Autodesk Fusion 360 part; units mm, degrees
(part 5 of 7)
  spline S636 degree 3 poles (-2.5533, 4.7746) (-2.5168, 4.7495) (-2.4648, 4.7165) (-2.4379, 4.7009) knots 0 0 0 0 1 1 1 1
  spline S637 degree 3 poles (-2.4379, 4.7009) (-2.4119, 4.6862) (-2.3824, 4.6662) (-2.3737, 4.6567) knots 0 0 0 0 1 1 1 1
  spline S638 degree 3 poles (-2.3737, 4.6567) (-2.359, 4.6393) (-2.359, 4.6385) (-2.3789, 4.622) knots 0 0 0 0 1 1 1 1
  spline S639 degree 3 poles (-2.3789, 4.622) (-2.391, 4.6116) (-2.3945, 4.6046) (-2.3884, 4.6038) knots 0 0 0 0 1 1 1 1
  spline S640 degree 3 poles (-2.3884, 4.6038) (-2.3824, 4.6038) (-2.3798, 4.5994) (-2.3832, 4.5942) knots 0 0 0 0 1 1 1 1
  spline S641 degree 3 poles (-2.3832, 4.5942) (-2.3867, 4.5873) (-2.4049, 4.5864) (-2.4353, 4.5899) knots 0 0 0 0 1 1 1 1
  line L91 (-2.4353, 4.5899) -> (-2.4821, 4.5951)
  line L92 (-2.4821, 4.5951) -> (-2.5411, 4.5413)
  spline S642 degree 3 poles (-2.5411, 4.5413) (-2.5732, 4.5118) (-2.6981, 4.3878) (-2.8187, 4.2663) knots 0 0 0 0 1 1 1 1
  spline S643 degree 3 poles (-2.8187, 4.2663) (-2.9661, 4.1171) (-3.0373, 4.0391) (-3.0373, 4.0261) knots 0 0 0 0 1 1 1 1
  spline S644 degree 3 poles (-3.0373, 4.0261) (-3.0373, 4.0018) (-2.9028, 3.8404) (-2.7875, 3.7277) knots 0 0 0 0 1 1 1 1
  spline S645 degree 3 poles (-2.7875, 3.7277) (-2.7363, 3.6773) (-2.6686, 3.608) (-2.6374, 3.5741) knots 0 0 0 0 1 1 1 1
  spline S646 degree 3 poles (-2.6374, 3.5741) (-2.6027, 3.5377) (-2.555, 3.4978) (-2.5168, 3.4752) knots 0 0 0 0 1 1 1 1
  line L93 (-2.5168, 3.4752) -> (-2.4535, 3.4379)
  line L94 (-2.4535, 3.4379) -> (-2.3485, 3.4379)
  spline S647 degree 3 poles (-2.3485, 3.4379) (-2.2774, 3.4388) (-2.228, 3.4431) (-2.1967, 3.4536) knots 0 0 0 0 1 1 1 1
  spline S648 degree 3 poles (-2.1967, 3.4536) (-2.1707, 3.4614) (-2.1308, 3.4674) (-2.1074, 3.4674) knots 0 0 0 0 1 1 1 1
  spline S649 degree 3 poles (-2.1074, 3.4674) (-2.0848, 3.4674) (-2.0432, 3.4752) (-2.0155, 3.4848) knots 0 0 0 0 1 1 1 1
  spline S650 degree 3 poles (-2.0155, 3.4848) (-1.9851, 3.4952) (-1.94, 3.503) (-1.901, 3.503) knots 0 0 0 0 1 1 1 1
  spline S651 degree 3 poles (-1.901, 3.503) (-1.8654, 3.5039) (-1.8012, 3.5099) (-1.7578, 3.5169) knots 0 0 0 0 1 1 1 1
  spline S652 degree 3 poles (-1.7578, 3.5169) (-1.6173, 3.5394) (-1.5904, 3.5412) (-1.5713, 3.5238) knots 0 0 0 0 1 1 1 1
  spline S653 degree 3 poles (-1.5713, 3.5238) (-1.5514, 3.5056) (-1.5488, 3.477) (-1.5653, 3.457) knots 0 0 0 0 1 1 1 1
  spline S654 degree 3 poles (-1.5653, 3.457) (-1.5705, 3.4501) (-1.6008, 3.4301) (-1.6321, 3.4137) knots 0 0 0 0 1 1 1 1
  spline S655 degree 3 poles (-1.6321, 3.4137) (-1.6633, 3.3972) (-1.7223, 3.3633) (-1.7639, 3.3391) knots 0 0 0 0 1 1 1 1
  spline S656 degree 3 poles (-1.7639, 3.3391) (-1.8047, 3.3156) (-1.848, 3.2931) (-1.8593, 3.2896) knots 0 0 0 0 1 1 1 1
  spline S657 degree 3 poles (-1.8593, 3.2896) (-1.8697, 3.2861) (-1.8992, 3.2705) (-1.9235, 3.2558) knots 0 0 0 0 1 1 1 1
  spline S658 degree 3 poles (-1.9235, 3.2558) (-1.9469, 3.241) (-1.9738, 3.2246) (-1.9816, 3.2202) knots 0 0 0 0 1 1 1 1
  spline S659 degree 3 poles (-1.9816, 3.2202) (-1.9894, 3.215) (-2.0224, 3.1933) (-2.0545, 3.1716) knots 0 0 0 0 1 1 1 1
  spline S660 degree 3 poles (-2.0545, 3.1716) (-2.0866, 3.1491) (-2.1525, 3.1109) (-2.2002, 3.0866) knots 0 0 0 0 1 1 1 1
  spline S661 degree 3 poles (-2.2002, 3.0866) (-2.3121, 3.0276) (-2.3555, 2.9938) (-2.4231, 2.9105) knots 0 0 0 0 1 1 1 1
  spline S662 degree 3 poles (-2.4231, 2.9105) (-2.4448, 2.8837) (-2.483, 2.8386) (-2.5081, 2.8108) knots 0 0 0 0 1 1 1 1
  spline S663 degree 3 poles (-2.5081, 2.8108) (-2.5342, 2.7813) (-2.5827, 2.7067) (-2.6244, 2.6312) knots 0 0 0 0 1 1 1 1
  spline S664 degree 3 poles (-2.6244, 2.6312) (-2.6704, 2.5471) (-2.7016, 2.4994) (-2.7137, 2.4951) knots 0 0 0 0 1 1 1 1
  spline S665 degree 3 poles (-2.7137, 2.4951) (-2.7397, 2.4855) (-2.8039, 2.5219) (-2.8707, 2.5835) knots 0 0 0 0 1 1 1 1
  spline S666 degree 3 poles (-2.8707, 2.5835) (-2.9002, 2.6122) (-2.9288, 2.6347) (-2.9341, 2.6347) knots 0 0 0 0 1 1 1 1
  spline S667 degree 3 poles (-2.9341, 2.6347) (-2.9384, 2.6347) (-2.9627, 2.6495) (-2.9878, 2.6677) knots 0 0 0 0 1 1 1 1
  spline S668 degree 3 poles (-2.9878, 2.6677) (-3.065, 2.7241) (-3.2134, 2.7882) (-3.3018, 2.8039) knots 0 0 0 0 1 1 1 1
  spline S669 degree 3 poles (-3.3018, 2.8039) (-3.3209, 2.8073) (-3.3426, 2.8134) (-3.3504, 2.8177) knots 0 0 0 0 1 1 1 1
  spline S670 degree 3 poles (-3.3504, 2.8177) (-3.3903, 2.8377) (-3.6306, 2.8706) (-3.7711, 2.875) knots 0 0 0 0 1 1 1 1
  spline S671 degree 3 poles (-3.7711, 2.875) (-3.9307, 2.8802) (-3.9602, 2.8767) (-3.9689, 2.855) knots 0 0 0 0 1 1 1 1
  spline S672 degree 3 poles (-3.9689, 2.855) (-3.9741, 2.842) (-3.8318, 2.554) (-3.739, 2.3901) knots 0 0 0 0 1 1 1 1
  spline S673 degree 3 poles (-3.739, 2.3901) (-3.7217, 2.358) (-3.7043, 2.3233) (-3.7009, 2.312) knots 0 0 0 0 1 1 1 1
  spline S674 degree 3 poles (-3.7009, 2.312) (-3.6974, 2.3007) (-3.6844, 2.2704) (-3.6731, 2.2444) knots 0 0 0 0 1 1 1 1
  spline S675 degree 3 poles (-3.6731, 2.2444) (-3.6054, 2.0978) (-3.5681, 1.9798) (-3.5837, 1.9642) knots 0 0 0 0 1 1 1 1
  spline S676 degree 3 poles (-3.5837, 1.9642) (-3.5924, 1.9546) (-3.6202, 1.9694) (-3.6662, 2.0058) knots 0 0 0 0 1 1 1 1
  spline S677 degree 3 poles (-3.6662, 2.0058) (-3.6852, 2.0214) (-3.713, 2.0405) (-3.7286, 2.0483) knots 0 0 0 0 1 1 1 1
  spline S678 degree 3 poles (-3.7286, 2.0483) (-3.7555, 2.0622) (-3.7572, 2.0622) (-3.7702, 2.0423) knots 0 0 0 0 1 1 1 1
  spline S679 degree 3 poles (-3.7702, 2.0423) (-3.7885, 2.0145) (-3.7997, 1.7239) (-3.8084, 1.069) knots 0 0 0 0 1 1 1 1
  spline S680 degree 3 poles (-3.8084, 1.069) (-3.8136, 0.6795) (-3.818, 0.5321) (-3.8266, 0.5095) knots 0 0 0 0 1 1 1 1
  spline S681 degree 3 poles (-3.8266, 0.5095) (-3.8657, 0.4011) (-3.9585, 0.2719) (-4.0322, 0.2224) knots 0 0 0 0 1 1 1 1
  spline S682 degree 3 poles (-4.0322, 0.2224) (-4.0999, 0.1773) (-4.2291, 0.0715) (-4.2907, 0.0108) knots 0 0 0 0 1 1 1 1
  spline S683 degree 3 poles (-4.2907, 0.0108) (-4.3566, -0.0534) (-4.3878, -0.076) (-4.511, -0.1454) knots 0 0 0 0 1 1 1 1
  spline S684 degree 3 poles (-4.511, -0.1454) (-4.5414, -0.1627) (-4.5822, -0.1887) (-4.7548, -0.3015) knots 0 0 0 0 1 1 1 1
  spline S685 degree 3 poles (-4.7548, -0.3015) (-4.8979, -0.3943) (-4.9309, -0.4143) (-4.9942, -0.442) knots 0 0 0 0 1 1 1 1
  spline S686 degree 3 poles (-4.9942, -0.442) (-5.028, -0.4568) (-5.0731, -0.4793) (-5.0939, -0.4915) knots 0 0 0 0 1 1 1 1
  spline S687 degree 3 poles (-5.0939, -0.4915) (-5.1147, -0.5045) (-5.172, -0.534) (-5.2214, -0.5583) knots 0 0 0 0 1 1 1 1
  spline S688 degree 3 poles (-5.2214, -0.5583) (-5.2709, -0.5834) (-5.3169, -0.6121) (-5.3247, -0.6233) knots 0 0 0 0 1 1 1 1
  spline S689 degree 3 poles (-5.3247, -0.6233) (-5.3437, -0.6537) (-5.3559, -0.6424) (-5.1191, -0.8168) knots 0 0 0 0 1 1 1 1
  spline S690 degree 3 poles (-5.1191, -0.8168) (-5.0558, -0.8627) (-4.9629, -0.9356) (-4.8693, -1.0111) knots 0 0 0 0 1 1 1 1
  spline S691 degree 3 poles (-4.8693, -1.0111) (-4.8441, -1.031) (-4.7895, -1.07) (-4.7478, -1.0969) knots 0 0 0 0 1 1 1 1
  spline S692 degree 3 poles (-4.7478, -1.0969) (-4.7062, -1.1238) (-4.655, -1.1594) (-4.6342, -1.175) knots 0 0 0 0 1 1 1 1
  spline S693 degree 3 poles (-4.6342, -1.175) (-4.6134, -1.1906) (-4.5622, -1.2253) (-4.5206, -1.2513) knots 0 0 0 0 1 1 1 1
  spline S694 degree 3 poles (-4.5206, -1.2513) (-4.4789, -1.2774) (-4.4156, -1.319) (-4.3809, -1.3433) knots 0 0 0 0 1 1 1 1
  spline S695 degree 3 poles (-4.3809, -1.3433) (-4.3453, -1.3676) (-4.2621, -1.4196) (-4.1953, -1.4595) knots 0 0 0 0 1 1 1 1
  spline S696 degree 3 poles (-4.1953, -1.4595) (-4.1285, -1.4994) (-4.06, -1.5428) (-4.0435, -1.5549) knots 0 0 0 0 1 1 1 1
  spline S697 degree 3 poles (-4.0435, -1.5549) (-4.027, -1.5679) (-3.994, -1.5888) (-3.9698, -1.6026) knots 0 0 0 0 1 1 1 1
  spline S698 degree 3 poles (-3.9698, -1.6026) (-3.9463, -1.6157) (-3.9151, -1.6365) (-3.9021, -1.6478) knots 0 0 0 0 1 1 1 1
  spline S699 degree 3 poles (-3.9021, -1.6478) (-3.8882, -1.6582) (-3.8726, -1.6677) (-3.8657, -1.6677) knots 0 0 0 0 1 1 1 1
  spline S700 degree 3 poles (-3.8657, -1.6677) (-3.8596, -1.6677) (-3.8414, -1.6798) (-3.8258, -1.6946) knots 0 0 0 0 1 1 1 1
  spline S701 degree 3 poles (-3.8258, -1.6946) (-3.8093, -1.7102) (-3.7867, -1.7267) (-3.7746, -1.7319) knots 0 0 0 0 1 1 1 1
  spline S702 degree 3 poles (-3.7746, -1.7319) (-3.7546, -1.7406) (-3.7355, -1.7536) (-3.6341, -1.8282) knots 0 0 0 0 1 1 1 1
  spline S703 degree 3 poles (-3.6341, -1.8282) (-3.5907, -1.8603) (-3.5673, -1.9132) (-3.5673, -1.9817) knots 0 0 0 0 1 1 1 1
  spline S704 degree 3 poles (-3.5673, -1.9817) (-3.5664, -2.0095) (-3.5612, -2.0737) (-3.5543, -2.1248) knots 0 0 0 0 1 1 1 1
  spline S705 degree 3 poles (-3.5543, -2.1248) (-3.5473, -2.176) (-3.5343, -2.2992) (-3.5265, -2.3981) knots 0 0 0 0 1 1 1 1
  line L95 (-3.5265, -2.3981) -> (-3.5109, -2.5768)
  line L96 (-3.5109, -2.5768) -> (-3.5395, -2.6609)
  spline S706 degree 3 poles (-3.5395, -2.6609) (-3.5551, -2.7069) (-3.5811, -2.7685) (-3.5976, -2.7971) knots 0 0 0 0 1 1 1 1
  spline S707 degree 3 poles (-3.5976, -2.7971) (-3.6141, -2.8257) (-3.6271, -2.85) (-3.6271, -2.8517) knots 0 0 0 0 1 1 1 1
  spline S708 degree 3 poles (-3.6271, -2.8517) (-3.6271, -2.8535) (-3.6419, -2.8795) (-3.6601, -2.909) knots 0 0 0 0 1 1 1 1
  spline S709 degree 3 poles (-3.6601, -2.909) (-3.7217, -3.0113) (-3.8206, -3.2221) (-3.8405, -3.2941) knots 0 0 0 0 1 1 1 1
  spline S710 degree 3 poles (-3.8405, -3.2941) (-3.8466, -3.3184) (-3.8605, -3.367) (-3.8709, -3.4025) knots 0 0 0 0 1 1 1 1
  spline S711 degree 3 poles (-3.8709, -3.4025) (-3.8804, -3.4381) (-3.896, -3.5006) (-3.9047, -3.5413) knots 0 0 0 0 1 1 1 1
  spline S712 degree 3 poles (-3.9047, -3.5413) (-3.9125, -3.5821) (-3.9238, -3.6324) (-3.9298, -3.6541) knots 0 0 0 0 1 1 1 1
  spline S713 degree 3 poles (-3.9298, -3.6541) (-3.9628, -3.7868) (-3.9914, -4.0991) (-3.9932, -4.335) knots 0 0 0 0 1 1 1 1
  spline S714 degree 3 poles (-3.9932, -4.335) (-3.994, -4.5198) (-3.9897, -4.5675) (-3.9724, -4.5892) knots 0 0 0 0 1 1 1 1
  spline S715 degree 3 poles (-3.9724, -4.5892) (-3.9385, -4.6299) (-3.7486, -4.6855) (-3.5248, -4.721) knots 0 0 0 0 1 1 1 1
  spline S716 degree 3 poles (-3.5248, -4.721) (-3.4666, -4.7297) (-3.4155, -4.7401) (-3.4111, -4.7427) knots 0 0 0 0 1 1 1 1
  spline S717 degree 3 poles (-3.4111, -4.7427) (-3.4068, -4.7453) (-3.3313, -4.7557) (-3.2437, -4.7661) knots 0 0 0 0 1 1 1 1
  spline S718 degree 3 poles (-3.2437, -4.7661) (-3.1041, -4.7826) (-3.0399, -4.7852) (-2.7077, -4.7852) knots 0 0 0 0 1 1 1 1
  spline S719 degree 3 poles (-2.7077, -4.7852) (-2.4561, -4.7861) (-2.3043, -4.7826) (-2.2523, -4.7757) knots 0 0 0 0 1 1 1 1
  spline S720 degree 3 poles (-2.2523, -4.7757) (-2.2098, -4.7696) (-2.1291, -4.7601) (-2.0744, -4.7549) knots 0 0 0 0 1 1 1 1
  spline S721 degree 3 poles (-2.0744, -4.7549) (-2.0198, -4.7496) (-1.9669, -4.741) (-1.9582, -4.7366) knots 0 0 0 0 1 1 1 1
  spline S722 degree 3 poles (-1.9582, -4.7366) (-1.9487, -4.7314) (-1.9105, -4.7236) (-1.8723, -4.7202) knots 0 0 0 0 1 1 1 1
  spline S723 degree 3 poles (-1.8723, -4.7202) (-1.835, -4.7158) (-1.796, -4.708) (-1.7865, -4.7028) knots 0 0 0 0 1 1 1 1
  spline S724 degree 3 poles (-1.7865, -4.7028) (-1.7778, -4.6976) (-1.7457, -4.6898) (-1.7162, -4.6855) knots 0 0 0 0 1 1 1 1
  spline S725 degree 3 poles (-1.7162, -4.6855) (-1.6468, -4.6751) (-1.5549, -4.6542) (-1.4881, -4.6334) knots 0 0 0 0 1 1 1 1
  spline S726 degree 3 poles (-1.4881, -4.6334) (-1.4594, -4.6247) (-1.4282, -4.6169) (-1.4187, -4.6169) knots 0 0 0 0 1 1 1 1
  spline S727 degree 3 poles (-1.4187, -4.6169) (-1.41, -4.6161) (-1.3866, -4.6091) (-1.3675, -4.5996) knots 0 0 0 0 1 1 1 1
  spline S728 degree 3 poles (-1.3675, -4.5996) (-1.3484, -4.59) (-1.3267, -4.5831) (-1.3198, -4.5822) knots 0 0 0 0 1 1 1 1
  spline S729 degree 3 poles (-1.3198, -4.5822) (-1.3128, -4.5822) (-1.2938, -4.5744) (-1.2781, -4.5649) knots 0 0 0 0 1 1 1 1
  spline S730 degree 3 poles (-1.2781, -4.5649) (-1.2625, -4.5553) (-1.2434, -4.5475) (-1.2348, -4.5475) knots 0 0 0 0 1 1 1 1
  spline S731 degree 3 poles (-1.2348, -4.5475) (-1.227, -4.5467) (-1.2044, -4.5397) (-1.1853, -4.5302) knots 0 0 0 0 1 1 1 1
  spline S732 degree 3 poles (-1.1853, -4.5302) (-1.1662, -4.5207) (-1.1446, -4.5128) (-1.1376, -4.5128) knots 0 0 0 0 1 1 1 1
  spline S733 degree 3 poles (-1.1376, -4.5128) (-1.1307, -4.5128) (-1.109, -4.505) (-1.0899, -4.4955) knots 0 0 0 0 1 1 1 1
  spline S734 degree 3 poles (-1.0899, -4.4955) (-1.0708, -4.486) (-1.0491, -4.4781) (-1.0422, -4.4781) knots 0 0 0 0 1 1 1 1
  spline S735 degree 3 poles (-1.0422, -4.4781) (-1.0353, -4.4781) (-1.0179, -4.4703) (-1.0032, -4.4608) knots 0 0 0 0 1 1 1 1
  spline S736 degree 3 poles (-1.0032, -4.4608) (-0.9893, -4.4513) (-0.9693, -4.4435) (-0.9607, -4.4435) knots 0 0 0 0 1 1 1 1
  spline S737 degree 3 poles (-0.9607, -4.4435) (-0.9416, -4.4435) (-0.9112, -4.4296) (-0.7273, -4.3385) knots 0 0 0 0 1 1 1 1
  spline S738 degree 3 poles (-0.7273, -4.3385) (-0.6519, -4.3003) (-0.5859, -4.27) (-0.5799, -4.27) knots 0 0 0 0 1 1 1 1
  spline S739 degree 3 poles (-0.5799, -4.27) (-0.5738, -4.27) (-0.5322, -4.2509) (-0.4871, -4.2275) knots 0 0 0 0 1 1 1 1
  spline S740 degree 3 poles (-0.4871, -4.2275) (-0.3578, -4.1607) (-0.3613, -4.1633) (-0.2251, -4.0731) knots 0 0 0 0 1 1 1 1
  spline S741 degree 3 poles (-0.2251, -4.0731) (-0.0906, -3.9837) (-0.0932, -3.9846) (0.1548, -3.9898) knots 0 0 0 0 1 1 1 1
  line L97 (0.1548, -3.9898) -> (0.3674, -3.9941)
  line L98 (0.3674, -3.9941) -> (0.4107, -4.021)
  spline S742 degree 3 poles (0.4107, -4.021) (0.4341, -4.0358) (0.4793, -4.0627) (0.5096, -4.0817) knots 0 0 0 0 1 1 1 1
  spline S743 degree 3 poles (0.5096, -4.0817) (0.5981, -4.1355) (0.6328, -4.1546) (0.697, -4.1841) knots 0 0 0 0 1 1 1 1
  spline S744 degree 3 poles (0.697, -4.1841) (0.7204, -4.1945) (0.7464, -4.2066) (0.7534, -4.211) knots 0 0 0 0 1 1 1 1
  spline S745 degree 3 poles (0.7534, -4.211) (0.7603, -4.2145) (0.7915, -4.2301) (0.8228, -4.2448) knots 0 0 0 0 1 1 1 1
  spline S746 degree 3 poles (0.8228, -4.2448) (0.8982, -4.2812) (0.9242, -4.2943) (0.9633, -4.3151) knots 0 0 0 0 1 1 1 1
  spline S747 degree 3 poles (0.9633, -4.3151) (0.9858, -4.3263) (0.9945, -4.3298) (1.0483, -4.3541) knots 0 0 0 0 1 1 1 1
  spline S748 degree 3 poles (1.0483, -4.3541) (1.1515, -4.4009) (1.1715, -4.4088) (1.1871, -4.4088) knots 0 0 0 0 1 1 1 1
  spline S749 degree 3 poles (1.1871, -4.4088) (1.1957, -4.4088) (1.2062, -4.4122) (1.2088, -4.4174) knots 0 0 0 0 1 1 1 1
  spline S750 degree 3 poles (1.2088, -4.4174) (1.2157, -4.4287) (1.2946, -4.466) (1.3441, -4.4816) knots 0 0 0 0 1 1 1 1
  spline S751 degree 3 poles (1.3441, -4.4816) (1.3649, -4.4886) (1.4039, -4.5024) (1.4299, -4.5128) knots 0 0 0 0 1 1 1 1
  spline S752 degree 3 poles (1.4299, -4.5128) (1.456, -4.5233) (1.4933, -4.5371) (1.5124, -4.5423) knots 0 0 0 0 1 1 1 1
  spline S753 degree 3 poles (1.5124, -4.5423) (1.5314, -4.5484) (1.5566, -4.5571) (1.5687, -4.5623) knots 0 0 0 0 1 1 1 1
  spline S754 degree 3 poles (1.5687, -4.5623) (1.5809, -4.5675) (1.6138, -4.5779) (1.6425, -4.5848) knots 0 0 0 0 1 1 1 1
  spline S755 degree 3 poles (1.6425, -4.5848) (1.6711, -4.5926) (1.7214, -4.6065) (1.7552, -4.6169) knots 0 0 0 0 1 1 1 1
  spline S756 degree 3 poles (1.7552, -4.6169) (1.8168, -4.6352) (1.927, -4.6594) (2.0467, -4.6811) knots 0 0 0 0 1 1 1 1
  spline S757 degree 3 poles (2.0467, -4.6811) (2.0831, -4.6881) (2.1204, -4.6967) (2.1291, -4.7019) knots 0 0 0 0 1 1 1 1
  spline S758 degree 3 poles (2.1291, -4.7019) (2.1386, -4.7063) (2.1725, -4.7132) (2.2063, -4.7158) knots 0 0 0 0 1 1 1 1
  spline S759 degree 3 poles (2.2063, -4.7158) (2.2392, -4.7193) (2.2861, -4.728) (2.3104, -4.734) knots 0 0 0 0 1 1 1 1
  spline S760 degree 3 poles (2.3104, -4.734) (2.3364, -4.7418) (2.4457, -4.7505) (2.588, -4.7557) knots 0 0 0 0 1 1 1 1
  spline S761 degree 3 poles (2.588, -4.7557) (2.9219, -4.7705) (3.1232, -4.78) (3.2082, -4.7861) knots 0 0 0 0 1 1 1 1
  spline S762 degree 3 poles (3.2082, -4.7861) (3.2489, -4.7896) (3.2836, -4.7896) (3.2862, -4.7869) knots 0 0 0 0 1 1 1 1
  spline S763 degree 3 poles (-0.2268, -3.6064) (-0.4333, -3.5838) (-0.7716, -3.5196) (-0.9858, -3.4624) knots 0 0 0 0 1 1 1 1
  spline S764 degree 3 poles (-0.9858, -3.4624) (-1.3285, -3.3696) (-1.6694, -3.2395) (-1.9053, -3.1102) knots 0 0 0 0 1 1 1 1
  spline S765 degree 3 poles (-1.9053, -3.1102) (-2.4891, -2.7901) (-2.8733, -2.4302) (-3.1882, -1.9071) knots 0 0 0 0 1 1 1 1
  spline S766 degree 3 poles (-3.1882, -1.9071) (-3.2611, -1.7874) (-3.4077, -1.4855) (-3.4519, -1.3641) knots 0 0 0 0 1 1 1 1
  spline S767 degree 3 poles (-3.4519, -1.3641) (-3.5864, -0.9989) (-3.6497, -0.73) (-3.6965, -0.3293) knots 0 0 0 0 1 1 1 1
  spline S768 degree 3 poles (-3.6965, -0.3293) (-3.7399, 0.0541) (-3.7659, 0.9025) (-3.7486, 1.403) knots 0 0 0 0 1 1 1 1
  spline S769 degree 3 poles (-3.7486, 1.403) (-3.7434, 1.5435) (-3.7373, 1.7283) (-3.7338, 1.8124) knots 0 0 0 0 1 1 1 1
  line L99 (-3.7338, 1.8124) -> (-3.7286, 1.9659)
  line L100 (-3.7286, 1.9659) -> (-3.6939, 1.9208)
  spline S770 degree 3 poles (-3.6939, 1.9208) (-3.674, 1.8957) (-3.6306, 1.8401) (-3.5959, 1.7976) knots 0 0 0 0 1 1 1 1
  spline S771 degree 3 poles (-3.5959, 1.7976) (-3.4606, 1.6268) (-3.2619, 1.3422) (-3.1327, 1.1341) knots 0 0 0 0 1 1 1 1
  spline S772 degree 3 poles (-3.1327, 1.1341) (-3.0286, 0.9649) (-2.9713, 0.8374) (-2.9514, 0.7299) knots 0 0 0 0 1 1 1 1
  spline S773 degree 3 poles (-2.9514, 0.7299) (-2.9445, 0.696) (-2.9358, 0.6743) (-2.9236, 0.6648) knots 0 0 0 0 1 1 1 1
  spline S774 degree 3 poles (-2.9236, 0.6648) (-2.908, 0.6526) (-2.9063, 0.6474) (-2.915, 0.6171) knots 0 0 0 0 1 1 1 1
  spline S775 degree 3 poles (-2.915, 0.6171) (-2.9193, 0.5989) (-2.9306, 0.5382) (-2.9393, 0.4835) knots 0 0 0 0 1 1 1 1
  spline S776 degree 3 poles (-2.9393, 0.4835) (-2.9618, 0.3395) (-2.9618, -0.1098) (-2.9393, -0.2538) knots 0 0 0 0 1 1 1 1
  spline S777 degree 3 poles (-2.9393, -0.2538) (-2.8733, -0.6745) (-2.7901, -0.9764) (-2.6357, -1.3554) knots 0 0 0 0 1 1 1 1
  spline S778 degree 3 poles (-2.6357, -1.3554) (-2.568, -1.5202) (-2.5628, -1.5272) (-2.5203, -1.5168) knots 0 0 0 0 1 1 1 1
  spline S779 degree 3 poles (-2.5203, -1.5168) (-2.4908, -1.509) (-2.4934, -1.4899) (-2.542, -1.3789) knots 0 0 0 0 1 1 1 1
  spline S780 degree 3 poles (-2.542, -1.3789) (-2.5862, -1.2756) (-2.6799, -1.0241) (-2.7241, -0.887) knots 0 0 0 0 1 1 1 1
  spline S781 degree 3 poles (-2.7241, -0.887) (-2.7823, -0.7057) (-2.8456, -0.3969) (-2.8638, -0.2018) knots 0 0 0 0 1 1 1 1
  spline S782 degree 3 poles (-2.8638, -0.2018) (-2.9202, 0.402) (-2.8239, 0.9077) (-2.5585, 1.403) knots 0 0 0 0 1 1 1 1
  spline S783 degree 3 poles (-2.5585, 1.403) (-2.5029, 1.5071) (-2.4127, 1.6415) (-2.3234, 1.7569) knots 0 0 0 0 1 1 1 1
  spline S784 degree 3 poles (-2.3234, 1.7569) (-2.2427, 1.8601) (-2.0371, 2.077) (-2.0328, 2.0639) knots 0 0 0 0 1 1 1 1
  spline S785 degree 3 poles (-2.0328, 2.0639) (-2.0311, 2.0587) (-2.0345, 2.0318) (-2.0397, 2.0041) knots 0 0 0 0 1 1 1 1
  spline S786 degree 3 poles (-2.0397, 2.0041) (-2.051, 1.9408) (-2.0701, 1.7283) (-2.0831, 1.5071) knots 0 0 0 0 1 1 1 1
  spline S787 degree 3 poles (-2.0831, 1.5071) (-2.0979, 1.2633) (-2.084, 0.9979) (-2.0389, 0.6509) knots 0 0 0 0 1 1 1 1
  spline S788 degree 3 poles (-2.0389, 0.6509) (-2.0233, 0.5347) (-2.0224, 0.5069) (-2.0311, 0.4124) knots 0 0 0 0 1 1 1 1
  spline S789 degree 3 poles (-2.0311, 0.4124) (-2.0423, 0.2918) (-2.0449, 0.0481) (-2.0354, -0.0378) knots 0 0 0 0 1 1 1 1
  line L101 (-2.0354, -0.0378) -> (-2.0293, -0.0951)
  line L102 (-2.0293, -0.0951) -> (-2.0753, -0.102)
  spline S790 degree 3 poles (-2.0753, -0.102) (-2.1013, -0.1055) (-2.1395, -0.1107) (-2.1612, -0.1142) knots 0 0 0 0 1 1 1 1
  line L103 (-2.1612, -0.1142) -> (-2.2002, -0.1194)
  line L104 (-2.2002, -0.1194) -> (-2.2028, -0.1783)
  line L105 (-2.2028, -0.1783) -> (-2.2054, -0.2365)
  line L106 (-2.2054, -0.2365) -> (-2.1551, -0.2321)
  spline S791 degree 3 poles (-2.1551, -0.2321) (-2.1273, -0.2287) (-2.0562, -0.2208) (-1.9964, -0.2139) knots 0 0 0 0 1 1 1 1
  spline S792 degree 3 poles (-1.9964, -0.2139) (-1.8307, -0.1931) (-1.8428, -0.187) (-1.7995, -0.3102) knots 0 0 0 0 1 1 1 1
  spline S793 degree 3 poles (-1.7995, -0.3102) (-1.7387, -0.4828) (-1.7119, -0.5453) (-1.6268, -0.7213) knots 0 0 0 0 1 1 1 1
  spline S794 degree 3 poles (-1.6268, -0.7213) (-1.5817, -0.8133) (-1.5453, -0.8905) (-1.5453, -0.8922) knots 0 0 0 0 1 1 1 1
  spline S795 degree 3 poles (-1.5453, -0.8922) (-1.5453, -0.894) (-1.5522, -0.8957) (-1.5609, -0.8957) knots 0 0 0 0 1 1 1 1
  spline S796 degree 3 poles (-1.5609, -0.8957) (-1.5791, -0.8957) (-1.9252, -0.9746) (-2.0397, -1.005) knots 0 0 0 0 1 1 1 1
  spline S797 degree 3 poles (-2.0397, -1.005) (-2.1794, -1.0423) (-2.1785, -1.0414) (-2.1785, -1.0674) knots 0 0 0 0 1 1 1 1
  spline S798 degree 3 poles (-2.1785, -1.0674) (-2.1785, -1.0805) (-2.1751, -1.0961) (-2.1707, -1.1021) knots 0 0 0 0 1 1 1 1
  spline S799 degree 3 poles (-2.1707, -1.1021) (-2.1612, -1.1178) (-2.1421, -1.1134) (-1.8012, -1.0293) knots 0 0 0 0 1 1 1 1
  spline S800 degree 3 poles (-1.8012, -1.0293) (-1.6581, -0.9937) (-1.5332, -0.9634) (-1.5228, -0.9608) knots 0 0 0 0 1 1 1 1
  spline S801 degree 3 poles (-1.5228, -0.9608) (-1.5071, -0.9573) (-1.4993, -0.9668) (-1.4716, -1.0197) knots 0 0 0 0 1 1 1 1
  spline S802 degree 3 poles (-1.4716, -1.0197) (-1.3458, -1.26) (-1.0526, -1.659) (-0.8661, -1.8429) knots 0 0 0 0 1 1 1 1
  spline S803 degree 3 poles (-0.8661, -1.8429) (-0.8427, -1.8663) (-0.8184, -1.8846) (-0.8123, -1.8846) knots 0 0 0 0 1 1 1 1
  spline S804 degree 3 poles (-0.8123, -1.8846) (-0.7846, -1.8846) (-0.7247, -1.7276) (-0.6467, -1.4508) knots 0 0 0 0 1 1 1 1
  spline S805 degree 3 poles (-0.6467, -1.4508) (-0.5495, -1.1091) (-0.5035, -0.9035) (-0.4003, -0.3536) knots 0 0 0 0 1 1 1 1
  spline S806 degree 3 poles (-0.4003, -0.3536) (-0.376, -0.2252) (-0.3509, -0.0925) (-0.3439, -0.0586) knots 0 0 0 0 1 1 1 1
  spline S807 degree 3 poles (-0.3439, -0.0586) (-0.3335, -0.0057) (-0.2962, 0.2311) (-0.2355, 0.6249) knots 0 0 0 0 1 1 1 1
  spline S808 degree 3 poles (-0.2355, 0.6249) (-0.226, 0.6856) (-0.2182, 0.7463) (-0.2182, 0.7593) knots 0 0 0 0 1 1 1 1
  spline S809 degree 3 poles (-0.2182, 0.7593) (-0.2182, 0.8036) (-0.2268, 0.8062) (-0.0533, 0.7012) knots 0 0 0 0 1 1 1 1
  spline S810 degree 3 poles (-0.0533, 0.7012) (0.141, 0.5833) (0.3717, 0.3499) (0.5365, 0.1062) knots 0 0 0 0 1 1 1 1
  spline S811 degree 3 poles (0.5365, 0.1062) (0.599, 0.0134) (0.7143, -0.1914) (0.7707, -0.3085) knots 0 0 0 0 1 1 1 1
  spline S812 degree 3 poles (0.7707, -0.3085) (0.821, -0.4134) (0.9355, -0.6823) (0.9355, -0.6962) knots 0 0 0 0 1 1 1 1
  spline S813 degree 3 poles (0.9355, -0.6962) (0.9355, -0.6997) (0.9026, -0.7005) (0.8618, -0.6979) knots 0 0 0 0 1 1 1 1
  spline S814 degree 3 poles (0.8618, -0.6979) (0.7915, -0.6936) (0.7881, -0.6945) (0.7881, -0.7118) knots 0 0 0 0 1 1 1 1
  spline S815 degree 3 poles (0.7881, -0.7118) (0.7881, -0.7569) (0.808, -0.7673) (0.9164, -0.7786) knots 0 0 0 0 1 1 1 1
  spline S816 degree 3 poles (0.9164, -0.7786) (0.9615, -0.7838) (0.9728, -0.7881) (0.9798, -0.8038) knots 0 0 0 0 1 1 1 1
  spline S817 degree 3 poles (0.9798, -0.8038) (0.9902, -0.8289) (1.083, -1.1568) (1.1255, -1.3216) knots 0 0 0 0 1 1 1 1
  spline S818 degree 3 poles (1.1255, -1.3216) (1.1576, -1.4456) (1.1992, -1.6486) (1.2218, -1.7952) knots 0 0 0 0 1 1 1 1
  spline S819 degree 3 poles (1.2218, -1.7952) (1.2278, -1.8299) (1.2348, -1.8603) (1.2391, -1.8629) knots 0 0 0 0 1 1 1 1
  spline S820 degree 3 poles (1.2391, -1.8629) (1.2686, -1.8811) (1.5705, -1.6009) (1.7171, -1.4179) knots 0 0 0 0 1 1 1 1
  spline S821 degree 3 poles (1.7171, -1.4179) (1.8159, -1.2947) (1.8654, -1.2227) (1.9417, -1.0926) knots 0 0 0 0 1 1 1 1
  spline S822 degree 3 poles (1.9417, -1.0926) (1.9816, -1.0232) (1.9998, -1.0007) (2.0103, -1.0033) knots 0 0 0 0 1 1 1 1
  spline S823 degree 3 poles (2.0103, -1.0033) (2.1074, -1.0319) (2.4075, -1.103) (2.4405, -1.1056) knots 0 0 0 0 1 1 1 1
  line L107 (2.4405, -1.1056) -> (2.4839, -1.1082)
  line L108 (2.4839, -1.1082) -> (2.4865, -1.0761)
  line L109 (2.4865, -1.0761) -> (2.4891, -1.0449)
  line L110 (2.4891, -1.0449) -> (2.4171, -1.0223)
  spline S824 degree 3 poles (2.4171, -1.0223) (2.3225, -0.9937) (2.2245, -0.9703) (2.1282, -0.9521) knots 0 0 0 0 1 1 1 1
  spline S825 degree 3 poles (2.1282, -0.9521) (2.0848, -0.9434) (2.0475, -0.9347) (2.0449, -0.9313) knots 0 0 0 0 1 1 1 1
  spline S826 degree 3 poles (2.0449, -0.9313) (2.0415, -0.9287) (2.0475, -0.907) (2.0588, -0.8827) knots 0 0 0 0 1 1 1 1
  spline S827 degree 3 poles (2.0588, -0.8827) (2.1421, -0.7031) (2.2523, -0.4099) (2.2852, -0.2807) knots 0 0 0 0 1 1 1 1
  line L111 (2.2852, -0.2807) -> (2.3008, -0.2174)
  line L112 (2.3008, -0.2174) -> (2.3884, -0.2226)
  spline S828 degree 3 poles (2.3884, -0.2226) (2.4362, -0.226) (2.4821, -0.2304) (2.4899, -0.233) knots 0 0 0 0 1 1 1 1
  spline S829 degree 3 poles (2.4899, -0.233) (2.5082, -0.2382) (2.5168, -0.2122) (2.5125, -0.1584) knots 0 0 0 0 1 1 1 1
  line L113 (2.5125, -0.1584) -> (2.5099, -0.1202)
  line L114 (2.5099, -0.1202) -> (2.4292, -0.1055)
  spline S830 degree 3 poles (2.4292, -0.1055) (2.385, -0.0977) (2.3468, -0.089) (2.3442, -0.0864) knots 0 0 0 0 1 1 1 1
  spline S831 degree 3 poles (2.3442, -0.0864) (2.3407, -0.0838) (2.3485, -0.0231) (2.3607, 0.0472) knots 0 0 0 0 1 1 1 1
  spline S832 degree 3 poles (2.3607, 0.0472) (2.4257, 0.4167) (2.4483, 0.6709) (2.4483, 1.0213) knots 0 0 0 0 1 1 1 1
  spline S833 degree 3 poles (2.4483, 1.0213) (2.4483, 1.3258) (2.4344, 1.4932) (2.3789, 1.8705) knots 0 0 0 0 1 1 1 1
  spline S834 degree 3 poles (2.3789, 1.8705) (2.3633, 1.9824) (2.3511, 2.0752) (2.3529, 2.0778) knots 0 0 0 0 1 1 1 1
  spline S835 degree 3 poles (2.3529, 2.0778) (2.3546, 2.0796) (2.3754, 2.0665) (2.3989, 2.0492) knots 0 0 0 0 1 1 1 1
  spline S836 degree 3 poles (2.3989, 2.0492) (2.4214, 2.0318) (2.4813, 1.9867) (2.5316, 1.9503) knots 0 0 0 0 1 1 1 1
  spline S837 degree 3 poles (2.5316, 1.9503) (2.6877, 1.8341) (2.8655, 1.658) (2.9757, 1.5114) knots 0 0 0 0 1 1 1 1
  spline S838 degree 3 poles (2.9757, 1.5114) (3.0702, 1.3856) (3.1171, 1.3093) (3.183, 1.1766) knots 0 0 0 0 1 1 1 1
  spline S839 degree 3 poles (3.183, 1.1766) (3.275, 0.9927) (3.3218, 0.8678) (3.3634, 0.7004) knots 0 0 0 0 1 1 1 1
  spline S840 degree 3 poles (3.3634, 0.7004) (3.4814, 0.2293) (3.4649, -0.331) (3.3166, -0.9235) knots 0 0 0 0 1 1 1 1
  spline S841 degree 3 poles (3.3166, -0.9235) (3.2923, -1.0206) (3.1969, -1.3051) (3.157, -1.3979) knots 0 0 0 0 1 1 1 1
  spline S842 degree 3 poles (3.157, -1.3979) (3.1422, -1.4326) (3.1301, -1.4691) (3.1301, -1.4777) knots 0 0 0 0 1 1 1 1
  spline S843 degree 3 poles (3.1301, -1.4777) (3.1301, -1.4951) (3.1639, -1.5081) (3.1856, -1.5003) knots 0 0 0 0 1 1 1 1
  spline S844 degree 3 poles (3.1856, -1.5003) (3.1978, -1.4951) (3.2906, -1.2713) (3.3201, -1.1724) knots 0 0 0 0 1 1 1 1
  spline S845 degree 3 poles (3.3201, -1.1724) (3.3938, -0.9304) (3.4606, -0.6294) (3.4918, -0.3935) knots 0 0 0 0 1 1 1 1
  spline S846 degree 3 poles (3.4918, -0.3935) (3.5109, -0.2469) (3.5144, -0.1896) (3.5152, 0.0151) knots 0 0 0 0 1 1 1 1
  spline S847 degree 3 poles (3.5152, 0.0151) (3.5161, 0.3135) (3.5013, 0.4401) (3.4328, 0.7238) knots 0 0 0 0 1 1 1 1
  spline S848 degree 3 poles (3.4328, 0.7238) (3.4042, 0.8426) (3.4016, 0.8938) (3.4207, 0.958) knots 0 0 0 0 1 1 1 1
  spline S849 degree 3 poles (3.4207, 0.958) (3.4667, 1.1115) (3.6627, 1.4455) (3.8943, 1.7629) knots 0 0 0 0 1 1 1 1
  spline S850 degree 3 poles (3.8943, 1.7629) (3.929, 1.8107) (3.9767, 1.8766) (4.001, 1.9104) knots 0 0 0 0 1 1 1 1
  line L115 (4.001, 1.9104) -> (4.0452, 1.9703)
  line L116 (4.0452, 1.9703) -> (4.0504, 1.8627)
  spline S851 degree 3 poles (4.0504, 1.8627) (4.0634, 1.599) (4.0686, 0.7654) (4.0591, 0.3968) knots 0 0 0 0 1 1 1 1
  spline S852 degree 3 poles (4.0591, 0.3968) (4.0409, -0.3353) (3.9862, -0.7205) (3.8362, -1.1698) knots 0 0 0 0 1 1 1 1
  spline S853 degree 3 poles (3.8362, -1.1698) (3.726, -1.5029) (3.6289, -1.7102) (3.4441, -2.006) knots 0 0 0 0 1 1 1 1
  spline S854 degree 3 poles (3.4441, -2.006) (3.1474, -2.4805) (2.7042, -2.8691) (2.1326, -3.1553) knots 0 0 0 0 1 1 1 1
  spline S855 degree 3 poles (2.1326, -3.1553) (2.0085, -3.2178) (1.6503, -3.3618) (1.521, -3.4017) knots 0 0 0 0 1 1 1 1
  spline S856 degree 3 poles (1.521, -3.4017) (1.3354, -3.4581) (1.0969, -3.517) (0.9225, -3.5491) knots 0 0 0 0 1 1 1 1
  spline S857 degree 3 poles (0.9225, -3.5491) (0.5738, -3.6125) (0.4003, -3.6289) (0.1158, -3.6237) knots 0 0 0 0 1 1 1 1
  spline S858 degree 3 poles (0.1158, -3.6237) (-0.0039, -3.6211) (-0.1574, -3.6133) (-0.2268, -3.6064) knots 0 0 0 0 1 1 1 1
  spline S859 degree 3 poles (-0.8705, -1.7354) (-0.8861, -1.7145) (-0.932, -1.659) (-0.9737, -1.6105) knots 0 0 0 0 1 1 1 1
  spline S860 degree 3 poles (-0.9737, -1.6105) (-1.0552, -1.515) (-1.109, -1.4439) (-1.2087, -1.299) knots 0 0 0 0 1 1 1 1
  spline S861 degree 3 poles (-1.2087, -1.299) (-1.3111, -1.1499) (-1.4299, -0.9512) (-1.4213, -0.9425) knots 0 0 0 0 1 1 1 1
  spline S862 degree 3 poles (-1.4213, -0.9425) (-1.4117, -0.933) (-0.6076, -0.7743) (-0.5669, -0.7743) knots 0 0 0 0 1 1 1 1
  spline S863 degree 3 poles (-0.5669, -0.7743) (-0.5599, -0.7743) (-0.5573, -0.7812) (-0.5608, -0.7942) knots 0 0 0 0 1 1 1 1
  spline S864 degree 3 poles (-0.5608, -0.7942) (-0.6172, -1.0518) (-0.7282, -1.4795) (-0.7698, -1.5983) knots 0 0 0 0 1 1 1 1
  spline S865 degree 3 poles (-0.7698, -1.5983) (-0.7872, -1.6486) (-0.808, -1.7076) (-0.8149, -1.731) knots 0 0 0 0 1 1 1 1
  spline S866 degree 3 poles (-0.8149, -1.731) (-0.8227, -1.7536) (-0.8314, -1.7718) (-0.8349, -1.7718) knots 0 0 0 0 1 1 1 1
  spline S867 degree 3 poles (-0.8349, -1.7718) (-0.8384, -1.7718) (-0.854, -1.7553) (-0.8705, -1.7354) knots 0 0 0 0 1 1 1 1
  spline S868 degree 3 poles (1.2747, -1.6703) (1.266, -1.6079) (1.2461, -1.5098) (1.2009, -1.3121) knots 0 0 0 0 1 1 1 1
  spline S869 degree 3 poles (1.2009, -1.3121) (1.1793, -1.2184) (1.1272, -1.0423) (1.0518, -0.8107) knots 0 0 0 0 1 1 1 1
  spline S870 degree 3 poles (1.0518, -0.8107) (1.0483, -0.7977) (1.0622, -0.7994) (1.2088, -0.8306) knots 0 0 0 0 1 1 1 1
  spline S871 degree 3 poles (1.2088, -0.8306) (1.2608, -0.8419) (1.3918, -0.8697) (1.4993, -0.8914) knots 0 0 0 0 1 1 1 1
  spline S872 degree 3 poles (1.4993, -0.8914) (1.6069, -0.913) (1.7457, -0.9425) (1.809, -0.9573) knots 0 0 0 0 1 1 1 1
  line L117 (1.809, -0.9573) -> (1.9226, -0.9833)
  line L118 (1.9226, -0.9833) -> (1.8836, -1.0501)
  spline S873 degree 3 poles (1.8836, -1.0501) (1.7682, -1.2453) (1.5661, -1.5003) (1.4282, -1.6243) knots 0 0 0 0 1 1 1 1
  spline S874 degree 3 poles (1.4282, -1.6243) (1.3935, -1.6556) (1.3493, -1.6955) (1.3302, -1.7128) knots 0 0 0 0 1 1 1 1
  spline S875 degree 3 poles (1.3302, -1.7128) (1.3111, -1.731) (1.2929, -1.7458) (1.2903, -1.7458) knots 0 0 0 0 1 1 1 1
  spline S876 degree 3 poles (1.2903, -1.7458) (1.2877, -1.7458) (1.2807, -1.7119) (1.2747, -1.6703) knots 0 0 0 0 1 1 1 1
  spline S877 degree 3 poles (1.7119, -0.8575) (1.4672, -0.802) (1.3259, -0.7725) (1.1827, -0.7482) knots 0 0 0 0 1 1 1 1
  spline S878 degree 3 poles (1.1827, -0.7482) (1.0179, -0.7196) (1.0179, -0.7196) (1.0058, -0.6771) knots 0 0 0 0 1 1 1 1
  spline S879 degree 3 poles (1.0058, -0.6771) (0.9928, -0.6311) (0.985, -0.6112) (0.9147, -0.449) knots 0 0 0 0 1 1 1 1
  spline S880 degree 3 poles (0.9147, -0.449) (0.8488, -0.2972) (0.7707, -0.141) (0.6935, -0.0066) knots 0 0 0 0 1 1 1 1
  spline S881 degree 3 poles (0.6935, -0.0066) (0.5139, 0.3048) (0.2667, 0.5815) (0.0291, 0.7368) knots 0 0 0 0 1 1 1 1
  spline S882 degree 3 poles (0.0291, 0.7368) (-0.062, 0.7966) (-0.2398, 0.886) (-0.2555, 0.8799) knots 0 0 0 0 1 1 1 1
  spline S883 degree 3 poles (-0.2555, 0.8799) (-0.2702, 0.8747) (-0.2771, 0.8417) (-0.3006, 0.6787) knots 0 0 0 0 1 1 1 1
  spline S884 degree 3 poles (-0.3006, 0.6787) (-0.3127, 0.5954) (-0.3726, 0.232) (-0.4073, 0.0324) knots 0 0 0 0 1 1 1 1
  spline S885 degree 3 poles (-0.4073, 0.0324) (-0.4133, -0.0049) (-0.4151, -0.0066) (-0.4437, -0.0066) knots 0 0 0 0 1 1 1 1
  spline S886 degree 3 poles (-0.4437, -0.0066) (-0.4732, -0.0066) (-0.474, -0.0057) (-0.4801, 0.0368) knots 0 0 0 0 1 1 1 1
  spline S887 degree 3 poles (-0.4801, 0.0368) (-0.4827, 0.0602) (-0.4862, 0.1305) (-0.4862, 0.1929) knots 0 0 0 0 1 1 1 1
  spline S888 degree 3 poles (-0.4862, 0.1929) (-0.4888, 0.4644) (-0.5105, 0.611) (-0.5747, 0.8071) knots 0 0 0 0 1 1 1 1
  spline S889 degree 3 poles (-0.5747, 0.8071) (-0.6527, 1.043) (-0.7516, 1.1818) (-0.9156, 1.2859) knots 0 0 0 0 1 1 1 1
  spline S890 degree 3 poles (-0.9156, 1.2859) (-1.109, 1.409) (-1.4152, 1.4064) (-1.6303, 1.2807) knots 0 0 0 0 1 1 1 1
  spline S891 degree 3 poles (-1.6303, 1.2807) (-1.7674, 1.2) (-1.9079, 1.0031) (-1.9521, 0.8305) knots 0 0 0 0 1 1 1 1
  spline S892 degree 3 poles (-1.9521, 0.8305) (-1.9608, 0.7949) (-1.9721, 0.7645) (-1.9773, 0.7628) knots 0 0 0 0 1 1 1 1
  spline S893 degree 3 poles (-1.9773, 0.7628) (-1.9868, 0.7602) (-1.9903, 0.8018) (-2.0059, 1.095) knots 0 0 0 0 1 1 1 1
  spline S894 degree 3 poles (-2.0059, 1.095) (-2.0155, 1.2781) (-2.012, 1.5591) (-1.9972, 1.6771) knots 0 0 0 0 1 1 1 1
  spline S895 degree 3 poles (-1.9972, 1.6771) (-1.992, 1.723) (-1.9842, 1.7387) (-1.9356, 1.8063) knots 0 0 0 0 1 1 1 1
  spline S896 degree 3 poles (-1.9356, 1.8063) (-1.8264, 1.9581) (-1.665, 2.109) (-1.4803, 2.2348) knots 0 0 0 0 1 1 1 1
  spline S897 degree 3 poles (-1.4803, 2.2348) (-1.2712, 2.3762) (-1.155, 2.4335) (-0.8887, 2.5245) knots 0 0 0 0 1 1 1 1
  spline S898 degree 3 poles (-0.8887, 2.5245) (-0.7056, 2.587) (-0.6276, 2.6069) (-0.4393, 2.6382) knots 0 0 0 0 1 1 1 1
  spline S899 degree 3 poles (-0.4393, 2.6382) (-0.1852, 2.6798) (-0.0577, 2.6894) (0.232, 2.6842) knots 0 0 0 0 1 1 1 1
  spline S900 degree 3 poles (0.232, 2.6842) (0.4983, 2.6798) (0.6545, 2.6668) (0.8496, 2.6295) knots 0 0 0 0 1 1 1 1
  spline S901 degree 3 poles (0.8496, 2.6295) (1.2495, 2.5549) (1.6607, 2.3771) (1.9374, 2.1585) knots 0 0 0 0 1 1 1 1
  spline S902 degree 3 poles (1.9374, 2.1585) (2.0814, 2.0449) (2.2505, 1.8731) (2.3034, 1.7872) knots 0 0 0 0 1 1 1 1
  spline S903 degree 3 poles (2.3034, 1.7872) (2.3399, 1.7274) (2.3572, 1.5157) (2.3642, 1.0681) knots 0 0 0 0 1 1 1 1
  spline S904 degree 3 poles (2.3642, 1.0681) (2.3711, 0.5902) (2.3581, 0.4315) (2.3251, 0.5841) knots 0 0 0 0 1 1 1 1
  spline S905 degree 3 poles (2.3251, 0.5841) (2.28, 0.7914) (2.2601, 0.8565) (2.2115, 0.9562) knots 0 0 0 0 1 1 1 1
  spline S906 degree 3 poles (2.2115, 0.9562) (2.0762, 1.2364) (1.8628, 1.3769) (1.5739, 1.3769) knots 0 0 0 0 1 1 1 1
  spline S907 degree 3 poles (1.5739, 1.3769) (1.1767, 1.3761) (0.9173, 1.0968) (0.8262, 0.572) knots 0 0 0 0 1 1 1 1
  spline S908 degree 3 poles (0.8262, 0.572) (0.808, 0.467) (0.8037, 0.4054) (0.7993, 0.2267) knots 0 0 0 0 1 1 1 1
  line L119 (0.7993, 0.2267) -> (0.7941, 0.0082)
  line L120 (0.7941, 0.0082) -> (0.7612, 0.003)
  spline S909 degree 3 poles (0.7612, 0.003) (0.7291, -0.0023) (0.7273, -0.004) (0.7325, -0.0265) knots 0 0 0 0 1 1 1 1
  spline S910 degree 3 poles (0.7325, -0.0265) (0.736, -0.0396) (0.7429, -0.0621) (0.7499, -0.0777) knots 0 0 0 0 1 1 1 1
  spline S911 degree 3 poles (0.7499, -0.0777) (0.7638, -0.1124) (0.7568, -0.1115) (1.1047, -0.1228) knots 0 0 0 0 1 1 1 1
  spline S912 degree 3 poles (1.1047, -0.1228) (1.2521, -0.128) (1.4473, -0.1376) (1.5384, -0.1454) knots 0 0 0 0 1 1 1 1
  spline S913 degree 3 poles (1.5384, -0.1454) (1.6286, -0.1523) (1.7561, -0.1619) (1.8203, -0.1671) knots 0 0 0 0 1 1 1 1
  spline S914 degree 3 poles (1.8203, -0.1671) (1.9409, -0.1757) (2.2219, -0.2035) (2.2262, -0.207) knots 0 0 0 0 1 1 1 1
  spline S915 degree 3 poles (2.2262, -0.207) (2.2314, -0.2104) (2.1751, -0.3917) (2.1326, -0.5088) knots 0 0 0 0 1 1 1 1
  spline S916 degree 3 poles (2.1326, -0.5088) (2.0623, -0.7023) (1.979, -0.8914) (1.9573, -0.9052) knots 0 0 0 0 1 1 1 1
  spline S917 degree 3 poles (1.9573, -0.9052) (1.9521, -0.9087) (1.9417, -0.9096) (1.9339, -0.9078) knots 0 0 0 0 1 1 1 1
  spline S918 degree 3 poles (1.9339, -0.9078) (1.9261, -0.9061) (1.8264, -0.8836) (1.7119, -0.8575) knots 0 0 0 0 1 1 1 1
  spline S919 degree 3 poles (-1.5115, -0.7942) (-1.639, -0.5244) (-1.7622, -0.2313) (-1.7622, -0.1957) knots 0 0 0 0 1 1 1 1
  spline S920 degree 3 poles (-1.7622, -0.1957) (-1.7622, -0.1809) (-1.776, -0.1827) (-1.1376, -0.141) knots 0 0 0 0 1 1 1 1
  spline S921 degree 3 poles (-1.1376, -0.141) (-0.9919, -0.1324) (-0.7794, -0.1202) (-0.6649, -0.115) knots 0 0 0 0 1 1 1 1
  spline S922 degree 3 poles (-0.6649, -0.115) (-0.4697, -0.1072) (-0.4558, -0.1055) (-0.4419, -0.0881) knots 0 0 0 0 1 1 1 1
  spline S923 degree 3 poles (-0.4419, -0.0881) (-0.4229, -0.0656) (-0.4229, -0.0725) (-0.4393, -0.1619) knots 0 0 0 0 1 1 1 1
  spline S924 degree 3 poles (-0.4393, -0.1619) (-0.5139, -0.5626) (-0.533, -0.6598) (-0.5391, -0.6754) knots 0 0 0 0 1 1 1 1
  spline S925 degree 3 poles (-0.5391, -0.6754) (-0.5452, -0.691) (-0.5599, -0.6953) (-0.6449, -0.7083) knots 0 0 0 0 1 1 1 1
  spline S926 degree 3 poles (-0.6449, -0.7083) (-0.8028, -0.7318) (-1.0162, -0.7725) (-1.207, -0.815) knots 0 0 0 0 1 1 1 1
  spline S927 degree 3 poles (-1.207, -0.815) (-1.4317, -0.8653) (-1.4421, -0.8671) (-1.4603, -0.8688) knots 0 0 0 0 1 1 1 1
  spline S928 degree 3 poles (-1.4603, -0.8688) (-1.4707, -0.8697) (-1.4855, -0.8471) (-1.5115, -0.7942) knots 0 0 0 0 1 1 1 1
  spline S929 degree 3 poles (2.0328, -0.0508) (2.005, -0.0326) (1.9695, 0.029) (1.9634, 0.0715) knots 0 0 0 0 1 1 1 1
  spline S930 degree 3 poles (1.9634, 0.0715) (1.9487, 0.1695) (2.0718, 0.2649) (2.1707, 0.232) knots 0 0 0 0 1 1 1 1
  spline S931 degree 3 poles (2.1707, 0.232) (2.2401, 0.2094) (2.2809, 0.1547) (2.2826, 0.0802) knots 0 0 0 0 1 1 1 1
  spline S932 degree 3 poles (2.2826, 0.0802) (2.2835, 0.0212) (2.2523, -0.0309) (2.1993, -0.0552) knots 0 0 0 0 1 1 1 1
  spline S933 degree 3 poles (2.1993, -0.0552) (2.156, -0.076) (2.0675, -0.0734) (2.0328, -0.0508) knots 0 0 0 0 1 1 1 1
  spline S934 degree 3 poles (1.9383, -0.0352) (1.9357, -0.0239) (1.9331, -0.0118) (1.9331, -0.0066) knots 0 0 0 0 1 1 1 1
  spline S935 degree 3 poles (1.9331, -0.0066) (1.9339, 0.0064) (1.9591, -0.03) (1.9591, -0.043) knots 0 0 0 0 1 1 1 1
  spline S936 degree 3 poles (1.9591, -0.043) (1.9591, -0.0621) (1.9443, -0.056) (1.9383, -0.0352) knots 0 0 0 0 1 1 1 1
  spline S937 degree 3 poles (-0.8687, -0.0109) (-0.8817, -0.0109) (-0.8852, -0.0049) (-0.8835, 0.0142) knots 0 0 0 0 1 1 1 1
  line L121 (-0.8835, 0.0142) -> (-0.8817, 0.0385)
  line L122 (-0.8817, 0.0385) -> (-0.854, 0.0168)
  spline S938 degree 3 poles (-0.854, 0.0168) (-0.8245, -0.0049) (-0.8158, -0.0257) (-0.8392, -0.0161) knots 0 0 0 0 1 1 1 1
  spline S939 degree 3 poles (-0.8392, -0.0161) (-0.847, -0.0135) (-0.86, -0.0109) (-0.8687, -0.0109) knots 0 0 0 0 1 1 1 1
  spline S940 degree 3 poles (-0.7724, 0.0108) (-0.8045, 0.0272) (-0.834, 0.0628) (-0.8548, 0.1096) knots 0 0 0 0 1 1 1 1
  spline S941 degree 3 poles (-0.8548, 0.1096) (-0.8696, 0.1417) (-0.8705, 0.1513) (-0.8618, 0.186) knots 0 0 0 0 1 1 1 1
  spline S942 degree 3 poles (-0.8618, 0.186) (-0.8349, 0.2857) (-0.7534, 0.33) (-0.6501, 0.3013) knots 0 0 0 0 1 1 1 1
  spline S943 degree 3 poles (-0.6501, 0.3013) (-0.5981, 0.2866) (-0.5695, 0.2562) (-0.553, 0.199) knots 0 0 0 0 1 1 1 1
  spline S944 degree 3 poles (-0.553, 0.199) (-0.5382, 0.1461) (-0.5417, 0.1148) (-0.5686, 0.0741) knots 0 0 0 0 1 1 1 1
  spline S945 degree 3 poles (-0.5686, 0.0741) (-0.6094, 0.0116) (-0.7126, -0.0205) (-0.7724, 0.0108) knots 0 0 0 0 1 1 1 1
  line L123 (2.2384, 0.245) -> (2.2063, 0.2666)
  line L124 (2.2063, 0.2666) -> (2.2384, 0.2666)
  spline S946 degree 3 poles (2.2384, 0.2666) (2.2644, 0.2666) (2.2696, 0.2632) (2.2731, 0.245) knots 0 0 0 0 1 1 1 1
  spline S947 degree 3 poles (2.2731, 0.245) (2.2757, 0.2328) (2.2757, 0.2233) (2.2739, 0.2233) knots 0 0 0 0 1 1 1 1
  spline S948 degree 3 poles (2.2739, 0.2233) (2.2722, 0.2233) (2.2557, 0.2328) (2.2384, 0.245) knots 0 0 0 0 1 1 1 1
  spline S949 degree 3 poles (1.9764, 0.2267) (1.9764, 0.2285) (1.9834, 0.2354) (1.9912, 0.2415) knots 0 0 0 0 1 1 1 1
  spline S950 degree 3 poles (1.9912, 0.2415) (2.005, 0.2528) (2.0059, 0.2519) (1.9946, 0.238) knots 0 0 0 0 1 1 1 1
  spline S951 degree 3 poles (1.9946, 0.238) (1.9834, 0.2241) (1.9764, 0.2198) (1.9764, 0.2267) knots 0 0 0 0 1 1 1 1
  spline S952 degree 3 poles (-0.5868, 0.3187) (-0.5894, 0.323) (-0.5885, 0.3274) (-0.5833, 0.3274) knots 0 0 0 0 1 1 1 1
  spline S953 degree 3 poles (-0.5833, 0.3274) (-0.5781, 0.3274) (-0.5764, 0.3343) (-0.579, 0.3421) knots 0 0 0 0 1 1 1 1
  spline S954 degree 3 poles (-0.579, 0.3421) (-0.5833, 0.3551) (-0.5825, 0.356) (-0.5747, 0.3447) knots 0 0 0 0 1 1 1 1
  spline S955 degree 3 poles (-0.5747, 0.3447) (-0.5695, 0.3378) (-0.5651, 0.3265) (-0.5651, 0.3204) knots 0 0 0 0 1 1 1 1
  spline S956 degree 3 poles (-0.5651, 0.3204) (-0.5651, 0.3083) (-0.579, 0.3065) (-0.5868, 0.3187) knots 0 0 0 0 1 1 1 1
  spline S957 degree 3 poles (-2.902, 0.8452) (-2.9358, 0.9528) (-3.0433, 1.1462) (-3.2064, 1.3917) knots 0 0 0 0 1 1 1 1
  spline S958 degree 3 poles (-3.2064, 1.3917) (-3.2663, 1.4802) (-3.3201, 1.5686) (-3.327, 1.5886) knots 0 0 0 0 1 1 1 1
  spline S959 degree 3 poles (-3.327, 1.5886) (-3.4441, 1.9113) (-3.4892, 2.0275) (-3.5777, 2.2314) knots 0 0 0 0 1 1 1 1
  spline S960 degree 3 poles (-3.5777, 2.2314) (-3.6462, 2.391) (-3.7217, 2.5428) (-3.8032, 2.6885) knots 0 0 0 0 1 1 1 1
  spline S961 degree 3 poles (-3.8032, 2.6885) (-3.8344, 2.7449) (-3.8613, 2.7978) (-3.8631, 2.8056) knots 0 0 0 0 1 1 1 1
  spline S962 degree 3 poles (-3.8631, 2.8056) (-3.8657, 2.8195) (-3.8561, 2.8212) (-3.7833, 2.8238) knots 0 0 0 0 1 1 1 1
  spline S963 degree 3 poles (-3.7833, 2.8238) (-3.6063, 2.8299) (-3.4302, 2.7995) (-3.2663, 2.7362) knots 0 0 0 0 1 1 1 1
  spline S964 degree 3 poles (-3.2663, 2.7362) (-3.0711, 2.6607) (-2.928, 2.5705) (-2.7614, 2.4161) knots 0 0 0 0 1 1 1 1
  spline S965 degree 3 poles (-2.7614, 2.4161) (-2.6721, 2.3328) (-2.6669, 2.3337) (-2.62, 2.4499) knots 0 0 0 0 1 1 1 1
  spline S966 degree 3 poles (-2.62, 2.4499) (-2.5559, 2.613) (-2.5194, 2.6798) (-2.4292, 2.7995) knots 0 0 0 0 1 1 1 1
  spline S967 degree 3 poles (-2.4292, 2.7995) (-2.3451, 2.9114) (-2.2523, 2.9877) (-2.1204, 3.0545) knots 0 0 0 0 1 1 1 1
  spline S968 degree 3 poles (-2.1204, 3.0545) (-2.0623, 3.0832) (-1.9278, 3.1326) (-1.9218, 3.1265) knots 0 0 0 0 1 1 1 1
  spline S969 degree 3 poles (-1.9218, 3.1265) (-1.9209, 3.1257) (-1.9235, 3.0892) (-1.9278, 3.0467) knots 0 0 0 0 1 1 1 1
  spline S970 degree 3 poles (-1.9278, 3.0467) (-1.933, 3.0034) (-1.9391, 2.8689) (-1.9417, 2.7466) knots 0 0 0 0 1 1 1 1
  spline S971 degree 3 poles (-1.9417, 2.7466) (-1.9461, 2.5289) (-1.9461, 2.5237) (-1.9278, 2.5055) knots 0 0 0 0 1 1 1 1
  spline S972 degree 3 poles (-1.9278, 2.5055) (-1.9027, 2.4803) (-1.8957, 2.482) (-1.8593, 2.5237) knots 0 0 0 0 1 1 1 1
  spline S973 degree 3 poles (-1.8593, 2.5237) (-1.7231, 2.6798) (-1.6225, 2.7605) (-1.4716, 2.8342) knots 0 0 0 0 1 1 1 1
  spline S974 degree 3 poles (-1.4716, 2.8342) (-1.3744, 2.8819) (-1.1897, 2.947) (-1.1532, 2.947) knots 0 0 0 0 1 1 1 1
  spline S975 degree 3 poles (-1.1532, 2.947) (-1.1394, 2.947) (-1.0353, 2.9079) (-1.0257, 2.8993) knots 0 0 0 0 1 1 1 1
  spline S976 degree 3 poles (-1.0257, 2.8993) (-1.024, 2.8975) (-1.0318, 2.8524) (-1.0422, 2.7995) knots 0 0 0 0 1 1 1 1
  spline S977 degree 3 poles (-1.0422, 2.7995) (-1.0535, 2.7414) (-1.0587, 2.6998) (-1.0535, 2.6946) knots 0 0 0 0 1 1 1 1
  spline S978 degree 3 poles (-1.0535, 2.6946) (-1.0422, 2.6833) (-0.9676, 2.7041) (-0.8358, 2.7553) knots 0 0 0 0 1 1 1 1
  spline S979 degree 3 poles (-0.8358, 2.7553) (-0.6892, 2.8117) (-0.6883, 2.8125) (-0.6154, 2.7952) knots 0 0 0 0 1 1 1 1
  spline S980 degree 3 poles (-0.6154, 2.7952) (-0.533, 2.777) (-0.4923, 2.757) (-0.4888, 2.7327) knots 0 0 0 0 1 1 1 1
  spline S981 degree 3 poles (-0.4888, 2.7327) (-0.4862, 2.7162) (-0.4931, 2.7128) (-0.5538, 2.6998) knots 0 0 0 0 1 1 1 1
  spline S982 degree 3 poles (-0.5538, 2.6998) (-0.6762, 2.6737) (-0.8453, 2.6278) (-0.9372, 2.5957) knots 0 0 0 0 1 1 1 1
  spline S983 degree 3 poles (-0.9372, 2.5957) (-1.2087, 2.5011) (-1.4846, 2.3502) (-1.6867, 2.1854) knots 0 0 0 0 1 1 1 1
  spline S984 degree 3 poles (-1.6867, 2.1854) (-1.7535, 2.1316) (-1.9304, 1.9581) (-1.9599, 1.9191) knots 0 0 0 0 1 1 1 1
  line L125 (-1.9599, 1.9191) -> (-1.9799, 1.8931)
  line L126 (-1.9799, 1.8931) -> (-1.9747, 1.9321)
  spline S985 degree 3 poles (-1.9747, 1.9321) (-1.9573, 2.0553) (-1.9539, 2.09) (-1.953, 2.1472) knots 0 0 0 0 1 1 1 1
  line L127 (-1.953, 2.1472) -> (-1.953, 2.2097)
  line L128 (-1.953, 2.2097) -> (-1.9868, 2.1923)
  spline S986 degree 3 poles (-1.9868, 2.1923) (-2.1239, 2.1229) (-2.4344, 1.7716) (-2.5767, 1.5253) knots 0 0 0 0 1 1 1 1
  spline S987 degree 3 poles (-2.5767, 1.5253) (-2.7051, 1.3023) (-2.83, 1.0074) (-2.8638, 0.8452) knots 0 0 0 0 1 1 1 1
  spline S988 degree 3 poles (-2.8638, 0.8452) (-2.869, 0.8183) (-2.8768, 0.7958) (-2.8803, 0.7958) knots 0 0 0 0 1 1 1 1
  spline S989 degree 3 poles (-2.8803, 0.7958) (-2.8837, 0.7958) (-2.8933, 0.8183) (-2.902, 0.8452) knots 0 0 0 0 1 1 1 1
  spline S990 degree 3 poles (2.1369, 0.8999) (2.1291, 0.9137) (2.1256, 0.9259) (2.1274, 0.9259) knots 0 0 0 0 1 1 1 1
  spline S991 degree 3 poles (2.1274, 0.9259) (2.13, 0.9259) (2.1378, 0.9137) (2.1456, 0.8999) knots 0 0 0 0 1 1 1 1
  spline S992 degree 3 poles (2.1456, 0.8999) (2.1534, 0.8851) (2.1568, 0.8738) (2.1551, 0.8738) knots 0 0 0 0 1 1 1 1
  spline S993 degree 3 poles (2.1551, 0.8738) (2.1525, 0.8738) (2.1447, 0.8851) (2.1369, 0.8999) knots 0 0 0 0 1 1 1 1
  spline S994 degree 3 poles (2.0979, 0.9814) (2.0979, 0.9918) (2.1022, 0.9875) (2.1143, 0.9606) knots 0 0 0 0 1 1 1 1
  spline S995 degree 3 poles (2.1143, 0.9606) (2.1239, 0.9398) (2.1239, 0.9398) (2.1117, 0.9554) knots 0 0 0 0 1 1 1 1
  spline S996 degree 3 poles (2.1117, 0.9554) (2.1039, 0.9649) (2.0979, 0.9762) (2.0979, 0.9814) knots 0 0 0 0 1 1 1 1
  spline S997 degree 3 poles (3.2524, 1.2165) (3.072, 1.5522) (2.8534, 1.8063) (2.5576, 2.0266) knots 0 0 0 0 1 1 1 1
  spline S998 degree 3 poles (2.5576, 2.0266) (2.4414, 2.1134) (2.2818, 2.2114) (2.2696, 2.2045) knots 0 0 0 0 1 1 1 1
  spline S999 degree 3 poles (2.2696, 2.2045) (2.2592, 2.1975) (2.267, 2.1021) (2.2852, 2.011) knots 0 0 0 0 1 1 1 1
  spline S1000 degree 3 poles (2.2852, 2.011) (2.293, 1.9763) (2.2974, 1.946) (2.2956, 1.9442) knots 0 0 0 0 1 1 1 1
  spline S1001 degree 3 poles (2.2956, 1.9442) (2.2939, 1.9425) (2.2392, 1.9928) (2.1751, 2.0561) knots 0 0 0 0 1 1 1 1
  spline S1002 degree 3 poles (2.1751, 2.0561) (1.992, 2.2357) (1.8411, 2.3424) (1.6078, 2.4569) knots 0 0 0 0 1 1 1 1
  spline S1003 degree 3 poles (1.6078, 2.4569) (1.3692, 2.574) (1.2131, 2.6286) (0.9667, 2.6824) knots 0 0 0 0 1 1 1 1
  spline S1004 degree 3 poles (0.9667, 2.6824) (0.906, 2.6963) (0.8496, 2.7128) (0.8427, 2.7197) knots 0 0 0 0 1 1 1 1
  spline S1005 degree 3 poles (0.8427, 2.7197) (0.8193, 2.744) (0.834, 2.7587) (0.9008, 2.7804) knots 0 0 0 0 1 1 1 1
  spline S1006 degree 3 poles (0.9008, 2.7804) (1.0092, 2.8143) (1.0405, 2.8117) (1.2027, 2.7501) knots 0 0 0 0 1 1 1 1
  spline S1007 degree 3 poles (1.2027, 2.7501) (1.2799, 2.7206) (1.3571, 2.6937) (1.3736, 2.6902) knots 0 0 0 0 1 1 1 1
  spline S1008 degree 3 poles (1.3736, 2.6902) (1.4039, 2.685) (1.4039, 2.685) (1.4039, 2.7162) knots 0 0 0 0 1 1 1 1
  spline S1009 degree 3 poles (1.4039, 2.7162) (1.4039, 2.7336) (1.3952, 2.7813) (1.3857, 2.8221) knots 0 0 0 0 1 1 1 1
  spline S1010 degree 3 poles (1.3857, 2.8221) (1.3753, 2.862) (1.3684, 2.8967) (1.3701, 2.8975) knots 0 0 0 0 1 1 1 1
  spline S1011 degree 3 poles (1.3701, 2.8975) (1.3718, 2.8993) (1.3996, 2.9114) (1.4308, 2.9244) knots 0 0 0 0 1 1 1 1
  line L129 (1.4308, 2.9244) -> (1.4889, 2.9478)
  line L130 (1.4889, 2.9478) -> (1.5635, 2.9305)
  spline S1012 degree 3 poles (1.5635, 2.9305) (1.7934, 2.8759) (1.9894, 2.7631) (2.1542, 2.5887) knots 0 0 0 0 1 1 1 1
  spline S1013 degree 3 poles (2.1542, 2.5887) (2.221, 2.5185) (2.2488, 2.4959) (2.2653, 2.4959) knots 0 0 0 0 1 1 1 1
  spline S1014 degree 3 poles (2.2653, 2.4959) (2.2774, 2.4959) (2.2896, 2.502) (2.2922, 2.5098) knots 0 0 0 0 1 1 1 1
  spline S1015 degree 3 poles (2.2922, 2.5098) (2.3026, 2.5376) (2.2974, 2.8637) (2.2835, 2.9912) knots 0 0 0 0 1 1 1 1
  spline S1016 degree 3 poles (2.2835, 2.9912) (2.2765, 3.0632) (2.2713, 3.1239) (2.2739, 3.1257) knots 0 0 0 0 1 1 1 1
  spline S1017 degree 3 poles (2.2739, 3.1257) (2.28, 3.1317) (2.3659, 3.1031) (2.4318, 3.0728) knots 0 0 0 0 1 1 1 1
  spline S1018 degree 3 poles (2.4318, 3.0728) (2.5272, 3.0294) (2.614, 2.9704) (2.6912, 2.8958) knots 0 0 0 0 1 1 1 1
  spline S1019 degree 3 poles (2.6912, 2.8958) (2.8187, 2.7735) (2.8933, 2.6529) (2.9809, 2.4343) knots 0 0 0 0 1 1 1 1
  spline S1020 degree 3 poles (2.9809, 2.4343) (2.9991, 2.3875) (3.0191, 2.3519) (3.026, 2.3511) knots 0 0 0 0 1 1 1 1
  spline S1021 degree 3 poles (3.026, 2.3511) (3.0329, 2.3493) (3.0841, 2.3892) (3.1388, 2.4395) knots 0 0 0 0 1 1 1 1
  spline S1022 degree 3 poles (3.1388, 2.4395) (3.3469, 2.6304) (3.556, 2.7397) (3.8067, 2.7908) knots 0 0 0 0 1 1 1 1
  spline S1023 degree 3 poles (3.8067, 2.7908) (3.8969, 2.8091) (4.223, 2.8273) (4.223, 2.8134) knots 0 0 0 0 1 1 1 1
  spline S1024 degree 3 poles (4.223, 2.8134) (4.223, 2.8108) (4.1979, 2.764) (4.1667, 2.7093) knots 0 0 0 0 1 1 1 1
  spline S1025 degree 3 poles (4.1667, 2.7093) (4.0955, 2.5827) (3.9975, 2.3858) (3.9203, 2.2114) knots 0 0 0 0 1 1 1 1